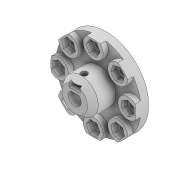
# Autodesk Inventor part: StepperWheelConnector
Saved by Autodesk Inventor 2022 (Build 260153000, 153)
## iProperties
Created: 2022-10-20
Part Number: StepperWheelConnector
Material: Generic
Document SubType Name: Modeling
Designer: MVeszpremi
Density: 1 g/cm^3
Appearance: Default
Author: MVeszpremi
Autodesk Inventor part; units mm, degrees
ref_plane "YZ Plane" through (0, 0, 0) normal (1, 0, 0) x (0, 1, 0)
ref_plane "XZ Plane" through (0, 0, 0) normal (0, 1, 0) x (-1, 0, 0)
ref_plane "XY Plane" through (0, 0, 0) normal (0, 0, 1) x (1, 0, 0)
sketch "Sketch1" plane through (0, 0, 0) normal (0, 0, 1) x (1, 0, 0)
  circle A0 centre (0, 0) radius 22.6275
  circle A1 centre (0, 0) radius 4.125
  line L0 (-2.6633, 3.15) -> (2.6633, 3.15)
  circle A2 centre (0, 0) radius 27.6275
  circle A3 centre (0, 22.6275) radius 2
  circle A4 centre (-16.0001, 16.0001) radius 2
  circle A5 centre (-22.6275, 0) radius 2
  circle A6 centre (-16.0001, -16.0001) radius 2
  circle A7 centre (0, -22.6275) radius 2
  circle A8 centre (16.0001, -16.0001) radius 2
  circle A9 centre (22.6275, 0) radius 2
  circle A10 centre (16.0001, 16.0001) radius 2
  circle A11 centre (0, 0) radius 11.25
  dimension "d0" = 45.255
  dimension "d1" = 8.25
  dimension "d2" = 3.15
  dimension "d3" = 5
  dimension "d4" = 4
  dimension "d7" = 360
  dimension "d11" = 22.5
  constraints: 11 centre point, 4 coincident, 2 end point, 2 point on circle, 1 horizontal, 1 vertical alignment, 19 other
  measures "d1" diameter of A1
  measures "d2" distance from line of point (0, 0) L0
  measures "d4" diameter of A3
  measures "d11" diameter of A11
extrude "Extrusion1" add sketch "Sketch1" against normal blind 5 contours A9 A0 A8 A7 A6 A5 A4 A3 A10 | L0 A1 | A2 | A11 picked at (-0.6202, 3.3272)
extrude "Extrusion2" add sketch "Sketch1" along normal blind 15.5 contours L0 A1 | A11 picked at (-0.6202, 3.3272)
sketch "Sketch3" plane through (0, 0, 0) normal (0, 0, 1) x (1, 0, 0)
  circle A0 centre (0, 22.6275) radius 2 projected
  line L0 (4.6188, 22.6275) -> (2.3094, 18.6275)
  line L1 (2.3094, 18.6275) -> (-2.3094, 18.6275)
  line L2 (-2.3094, 18.6275) -> (-4.6188, 22.6275)
  line L3 (-4.6188, 22.6275) -> (-2.3094, 26.6275)
  line L4 (-2.3094, 26.6275) -> (2.3094, 26.6275)
  line L5 (2.3094, 26.6275) -> (4.6188, 22.6275)
  circle A1 centre (0, 22.6275) radius 6.5
  circle A2 centre (0, 0) radius 11.25 projected
  circle A3 centre (0, 0) radius 27.6275 projected
  circle A4 centre (0, 22.6275) radius 2 projected
  circle A5 centre (-16.0001, 16.0001) radius 2 projected
  circle A6 centre (-22.6275, 0) radius 2 projected
  circle A7 centre (-16.0001, -16.0001) radius 2 projected
  circle A8 centre (0, -22.6275) radius 2 projected
  circle A9 centre (16.0001, -16.0001) radius 2 projected
  circle A10 centre (22.6275, 0) radius 2 projected
  circle A11 centre (16.0001, 16.0001) radius 2 projected
  point P0 (4.5734, 27.2463)
  point P1 (-4.5734, 27.2463)
  dimension "d15" = 8
  dimension "d16" = 13
  constraints: 12 end point, 2 coincident, 1 centre point, 13 other
  measures "d15" distance between parallel lines of L1 L4
  measures "d16" diameter of A1
extrude "Extrusion3" add sketch "Sketch3" along normal blind 3.5 contours A1 A3 picked at (-4.1626, 25.0833)
pattern_circular "Circular Pattern1" count 8 over 360 about axis through (0, 0, 0) along (0, 0, -1) of "Extrusion3"
sketch "Sketch4" plane through (0, 0, 15.5) normal (0, 0, 1) x (1, 0, 0)
  line L0 (-3.5, 8.4) -> (3.5, 8.4)
  line L1 (3.5, 8.4) -> (3.5, 4.9)
  line L2 (3.5, 4.9) -> (-3.5, 4.9)
  line L3 (-3.5, 4.9) -> (-3.5, 8.4)
  line L4 (2.6633, 3.15) -> (-2.6633, 3.15) projected
  line L5 (0, 3.15) -> (0, 11.4081)
  point P0 (0, 0)
  point P1 (0, 8.4)
  dimension "d22" = 7
  dimension "d23" = 3.5
  dimension "d24" = 1.75
  constraints: 10 end point, 2 midpoint, 2 parallel, 1 horizontal, 1 perpendicular, 1 point on line, 1 vertical
  measures "d22" distance of L0.start L0.end
  measures "d23" distance of L0.end L1.end
  measures "d24" distance between parallel lines of L4 L2
extrude "Extrusion4" cut sketch "Sketch4" against normal blind 10
sketch "Sketch5" plane through (-3.5, 4.9, 15.5) normal (0, 1, 0) x (1, 0, 0)
  line L0 (0.8367, 0) -> (6.1633, 0) projected
  line L1 (0, 10) -> (7, 10) projected
  circle A0 centre (3.5, 6.05) radius 2
  line L2 (7, 0) -> (7, 10) projected
  line L3 (7, 10) -> (0.8367, 0)
  point P0 (3.5, 15.5)
  dimension "d27" = 4
  dimension "d32" = 3.95
  constraints: 2 end point, 1 centre point
  measures "d27" diameter of A0
  measures "d32" distance from line of A0.centre L1
extrude "Extrusion5" cut sketch "Sketch5" along normal blind 10 and the other way blind 3
chamfer "Chamfer1" distance 3 distance2 4 1 edges at (-11.25, 0, 15.5) measured on face at (-10.75, 0, 15.5)
body "Solid1"
